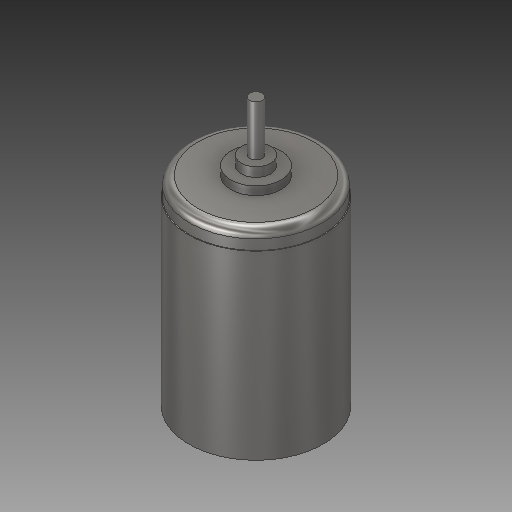
# Autodesk Inventor part: Motor
Saved by Autodesk Inventor 2019 (Build 230136000, 136)
## iProperties
Part Number: Motor
Material: Acero inoxidable
Document SubType Name: Modeling
Designer: carlos
Density: 8 g/cm^3
Appearance: Semipulido
Author: carlos
Autodesk Inventor part; units mm, degrees
ref_plane "YZ Plane" through (0, 0, 0) normal (1, 0, 0) x (0, 1, 0)
ref_plane "XZ Plane" through (0, 0, 0) normal (0, 1, 0) x (-1, 0, 0)
ref_plane "XY Plane" through (0, 0, 0) normal (0, 0, 1) x (1, 0, 0)
sketch "Boceto1" plane through (0, 0, 0) normal (0, 1, 0) x (-1, 0, 0)
  circle A0 centre (0, 0) radius 8
  dimension "d0" = 16
  constraints: 1 centre point, 1 coincident
  measures "d0" diameter of A0
extrude "Extrusión1" add sketch "Boceto1" along normal blind 21.6
sketch "Boceto2" plane through (0, 21.6, 0) normal (0, 1, 0) x (1, 0, 0)
  circle A0 centre (0, 0) radius 7.9
  dimension "d3" = 15.8
  constraints: 1 centre point, 1 coincident
  measures "d3" diameter of A0
extrude "Extrusión2" add sketch "Boceto2" along normal blind 2.2
fillet "Empalme1" radius 1 1 edges at (-7.9, 23.8, 0)
sketch "Boceto3" plane through (0, 23.8, 0) normal (0, 1, 0) x (1, 0, 0)
  circle A0 centre (0, 0) radius 3
  circle A1 centre (0, 0) radius 1.75
  circle A2 centre (0, 0) radius 0.75
  dimension "d7" = 6
  dimension "d8" = 3.5
  dimension "d13" = 1.5
  constraints: 3 centre point, 3 coincident
  measures "d7" diameter of A0
  measures "d8" diameter of A1
  measures "d13" diameter of A2
extrude "Extrusión3" add sketch "Boceto3" along normal blind 1 contours A0
extrude "Extrusión4" add sketch "Boceto3" along normal blind 2.1 contours A1 | A2
extrude "Extrusión5" add sketch "Boceto3" along normal blind 8.1 contours A2
sketch "Boceto4" plane through (0, 0, 0) normal (0, -1, 0) x (1, 0, 0)
  circle A0 centre (0, 0) radius 0.75 projected
  circle A1 centre (0, 0) radius 6.5
  dimension "d16" = 13
  constraints: 1 centre point, 1 coincident
  measures "d16" diameter of A1
extrude "Extrusión6" add sketch "Boceto4" along normal blind 1 contours A0 | A1
